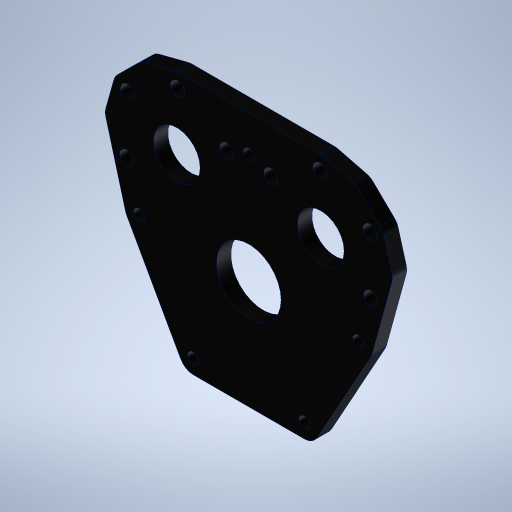
# Autodesk Inventor part: BottomPlate_Gearboxes_2_Exercise_2
Saved by Autodesk Inventor 2024 (Build 280153000, 153)
## iProperties
Created: 2024-11-16
Part Number: BottomPlate_Gearboxes_2_Exercise_2
Material: Aluminum 6061
Document SubType Name: Modeling
Designer: Danielle
Density: 2.7 g/cm^3
Appearance: Aluminum - Flat
Author: Danielle
Autodesk Inventor part; units mm, degrees
ref_plane "YZ Plane" through (0, 0, 0) normal (1, 0, 0) x (0, 1, 0)
ref_plane "XZ Plane" through (0, 0, 0) normal (0, 1, 0) x (-1, 0, 0)
ref_plane "XY Plane" through (0, 0, 0) normal (0, 0, 1) x (1, 0, 0)
sketch "Sketch1" plane through (0, 0, 0) normal (0, 0, 1) x (1, 0, 0)
  circle A0 centre (0, 0) radius 38.1 construction
  circle A1 centre (0, 0) radius 40.64 construction
  circle A2 centre (0, 0) radius 14.2875
  circle A3 centre (-31.9157, 32.7369) radius 30.0609 construction
  circle A4 centre (-31.9157, 32.7369) radius 25.4 construction
  circle A5 centre (-31.9157, 32.7369) radius 7.62 construction
  circle A6 centre (-53.7497, 45.7153) radius 3.175
  circle A7 centre (-57.3137, 33.0595) radius 3.175 construction
  circle A8 centre (-54.0723, 20.3173) radius 3.175
  circle A9 centre (-44.8941, 10.903) radius 3.175 construction
  circle A10 centre (-32.2383, 7.339) radius 3.175 construction
  circle A11 centre (-19.4961, 10.5803) radius 3.175 construction
  circle A12 centre (-10.0817, 19.7586) radius 3.175 construction
  circle A13 centre (-6.5178, 32.4143) radius 3.175 construction
  circle A14 centre (-9.7591, 45.1565) radius 3.175
  circle A15 centre (-18.9373, 54.5709) radius 3.175 construction
  circle A16 centre (-31.5931, 58.1349) radius 3.175
  circle A17 centre (-44.3353, 54.8935) radius 3.175 construction
  line L0 (-54.0723, 20.3173) -> (0, 0) construction
  line L1 (0, 0) -> (-18.9373, 54.5709) construction
  circle A18 centre (-48.5745, 1.2342) radius 2.4892
  circle A19 centre (-48.5745, 1.2342) radius 6.35 construction
  circle A20 centre (-48.5745, 1.2342) radius 3.9751 construction
  line L2 (-46.7163, 4.7482) -> (-45.9682, 6.1628) construction
  line L3 (-42.2266, 1.0729) -> (-40.6269, 1.0322) construction
  circle A21 centre (0, 48.5902) radius 6.35 construction
  circle A22 centre (0, 48.5902) radius 3.9751 construction
  circle A23 centre (0, 48.5902) radius 2.4892
  line L4 (0, 42.2402) -> (0, 40.64) construction
  line L5 (-3.5601, 46.8218) -> (-4.9932, 46.1099) construction
  circle A24 centre (-24.6505, -41.8731) radius 6.35 construction
  circle A25 centre (-24.6505, -41.8731) radius 2.4892
  line L6 (-21.4291, -36.4009) -> (-20.6173, -35.022)
  line L7 (0, 48.5902) -> (0, 0) construction
  circle A26 centre (31.9157, 32.7369) radius 30.0609 construction
  circle A27 centre (31.9157, 32.7369) radius 25.4 construction
  circle A28 centre (53.7497, 45.7153) radius 3.175
  circle A29 centre (57.3137, 33.0595) radius 3.175 construction
  circle A30 centre (54.0723, 20.3173) radius 3.175
  circle A31 centre (44.8941, 10.903) radius 3.175 construction
  circle A32 centre (9.7591, 45.1565) radius 3.175
  circle A33 centre (18.9373, 54.5709) radius 3.175 construction
  circle A34 centre (31.5931, 58.1349) radius 3.175
  circle A35 centre (44.3353, 54.8935) radius 3.175 construction
  circle A36 centre (48.5745, 1.2342) radius 2.4892
  circle A37 centre (48.5745, 1.2342) radius 6.35 construction
  circle A38 centre (48.5745, 1.2342) radius 3.9751 construction
  circle A39 centre (0, 48.5902) radius 2.4892 construction
  circle A40 centre (24.6505, -41.8731) radius 6.35 construction
  circle A41 centre (24.6505, -41.8731) radius 2.4892
  circle A42 centre (31.9157, 32.7369) radius 7.62 construction
  line L8 (-48.5745, 1.2342) -> (-24.6505, -41.8731) construction
  line L9 (24.6505, -41.8731) -> (-24.6505, -41.8731) construction
  circle A43 centre (-31.9157, 32.7369) radius 10.3188
  circle A44 centre (31.9157, 32.7369) radius 10.3188
  line L10 (-54.1268, -1.8472) -> (-30.2028, -44.9545)
  line L11 (-24.6505, -48.2231) -> (24.6505, -48.2231)
  line L12 (30.2028, -44.9545) -> (54.1268, -1.8472)
  circle A45 centre (44.3353, 54.8935) radius 6.35 construction
  circle A46 centre (53.7497, 45.7153) radius 6.35 construction
  circle A47 centre (31.5931, 58.1349) radius 6.35 construction
  circle A48 centre (57.3137, 33.0595) radius 6.35 construction
  circle A49 centre (54.0723, 20.3173) radius 6.35 construction
  circle A50 centre (-54.0723, 20.3173) radius 6.35 construction
  circle A51 centre (-57.3137, 33.0595) radius 6.35 construction
  circle A52 centre (-53.7497, 45.7153) radius 6.35 construction
  circle A53 centre (-44.3353, 54.8935) radius 6.35 construction
  circle A54 centre (-31.5931, 58.1349) radius 6.35 construction
  line L13 (-63.4259, 34.7808) -> (-59.8619, 47.4366)
  line L14 (-58.1824, 50.2621) -> (-48.768, 59.4403)
  line L15 (-45.9008, 61.0475) -> (-33.1586, 64.2889)
  line L16 (63.4259, 34.7808) -> (59.8619, 47.4366)
  line L17 (58.1824, 50.2621) -> (48.768, 59.4403)
  line L18 (45.9008, 61.0475) -> (33.1586, 64.2889)
  line L19 (-63.437, 31.3781) -> (-54.6979, -0.4473)
  line L20 (63.437, 31.3781) -> (54.6979, -0.4473)
  line L21 (-31.5931, 64.4849) -> (31.5931, 64.4849)
  arc A55 (-30.2028, -44.9545) -> (-24.6505, -48.2231) centre (-24.6505, -41.8731) ccw
  arc A56 (-54.6979, -0.4473) -> (-54.1268, -1.8472) centre (-48.5745, 1.2342) ccw
  arc A57 (-63.4259, 34.7808) -> (-63.437, 31.3781) centre (-57.3137, 33.0595) ccw
  arc A58 (-58.1824, 50.2621) -> (-59.8619, 47.4366) centre (-53.7497, 45.7153) ccw
  arc A59 (-45.9008, 61.0475) -> (-48.768, 59.4403) centre (-44.3353, 54.8935) ccw
  arc A60 (-31.5931, 64.4849) -> (-33.1586, 64.2889) centre (-31.5931, 58.1349) ccw
  arc A61 (33.1586, 64.2889) -> (31.5931, 64.4849) centre (31.5931, 58.1349) ccw
  arc A62 (48.768, 59.4403) -> (45.9008, 61.0475) centre (44.3353, 54.8935) ccw
  arc A63 (59.8619, 47.4366) -> (58.1824, 50.2621) centre (53.7497, 45.7153) ccw
  arc A64 (63.437, 31.3781) -> (63.4259, 34.7808) centre (57.3137, 33.0595) ccw
  arc A65 (54.1268, -1.8472) -> (54.6979, -0.4473) centre (48.5745, 1.2342) ccw
  arc A66 (24.6505, -48.2231) -> (30.2028, -44.9545) centre (24.6505, -41.8731) ccw
  dimension "d4" = 50.8
  dimension "d15" = 7.9502
  dimension "d22" = 12.7
  dimension "d0" = 76.2
  dimension "d1" = 2.54
  dimension "d2" = 28.575
  dimension "d3" = 60.1218
  dimension "d5" = 15.24
  dimension "d6" = 6.35
  dimension "d9" = 360
  dimension "d12" = 12.7
  dimension "d14" = 4.9784
  dimension "d16" = 1.6002
  dimension "d17" = 15.24
  dimension "d18" = 20.6375
  dimension "d19" = 20.6375
  dimension "d20" = 12.7
  dimension "d21" = 12.7
  dimension "d23" = 12.7
  dimension "d24" = 12.7
  dimension "d25" = 12.7
  dimension "d26" = 12.7
  dimension "d27" = 12.7
  dimension "d28" = 12.7
  dimension "d29" = 12.7
  constraints: 60 centre point, 45 point on circle, 44 end point, 25 coincident, 23 symmetric about line, 18 tangent, 10 point on line, 9 concentric, 6 equal length, 3 equal radius, 3 horizontal, 3 vertical, 2 vertical alignment, 63 other
  measures "d0" diameter of A0
  measures "d1" radial gap between concentric circles of A1 A0
  measures "d2" diameter of A2
  measures "d3" diameter of A3
  measures "d5" diameter of A5
  measures "d6" diameter of A6
  measures "d12" diameter of A19
  measures "d14" diameter of A18
  measures "d16" distance of L2.start L2.end
  measures "d17" diameter of A42
  measures "d18" diameter of A43
  measures "d19" diameter of A44
  measures "d20" diameter of A45
  measures "d21" diameter of A46
  measures "d23" diameter of A48
  measures "d24" diameter of A49
  measures "d25" diameter of A50
  measures "d26" diameter of A51
  measures "d27" diameter of A52
  measures "d28" diameter of A53
  measures "d29" diameter of A54
extrude "Extrusion1" add sketch "Sketch1" along normal blind 6.35
body "Solid1"
